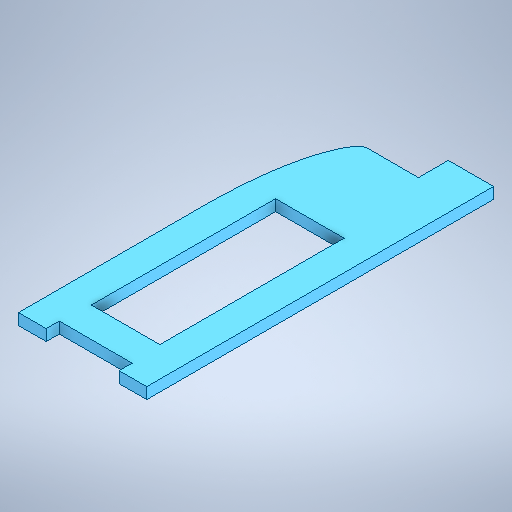
# Autodesk Inventor part: C-D
Saved by Autodesk Inventor 2025.3 (Build 293356030, 356C)
## iProperties
Created: 2025-07-09
Part Number: C-D
Material: Generic
Document SubType Name: Modeling
Designer: jv
Density: 1 g/cm^3
Appearance: Default(1)
Author: jv
Autodesk Inventor part; units mm, degrees
ref_plane "YZ Plane" through (0, 0, 0) normal (1, 0, 0) x (0, 1, 0)
ref_plane "XZ Plane" through (0, 0, 0) normal (0, 1, 0) x (-1, 0, 0)
ref_plane "XY Plane" through (0, 0, 0) normal (0, 0, 1) x (1, 0, 0)
sketch "Sketch1" plane through (0, 0, 0) normal (0, 1, 0) x (-1, 0, 0)
  line L0 (25.8082, 8) -> (28.6076, 7.9624) construction
  line L1 (0, 0) -> (0, 92.83)
  line L2 (0, 0) -> (12.1, 0)
  line L3 (26.34, 81.33) -> (8, 81.33)
  line L4 (8, 81.33) -> (8, 32)
  line L5 (8, 32) -> (26.34, 32)
  line L6 (26.34, 32) -> (26.34, 81.33)
  line L7 (0, 92.83) -> (7.42, 92.83)
  line L8 (7.42, 92.83) -> (7.42, 89.33)
  line L9 (7.42, 89.33) -> (26.92, 89.33)
  line L10 (26.92, 89.33) -> (26.92, 92.83)
  line L11 (26.92, 92.83) -> (34.34, 92.83)
  line L12 (34.34, 92.83) -> (34.34, 0)
  line L13 (34.34, 0) -> (12.1, 0)
  line L14 (12.1, 0) -> (12.1, 8)
  line L15 (12.1, 8) -> (34.34, 8)
  spline S0 degree 3 poles (25.8082, 8) (28.6076, 7.9624) (34.5101, 18.742) (34.34, 45.0104) knots 1 1 1 1 1.641396 1.641396 1.641396 1.641396
  line L16 (28.6076, 7.9624) -> (34.5101, 18.742) construction
  line L17 (34.5101, 18.742) -> (34.34, 45.0104) construction
  point P0 (25.8768, 44.3592)
  point P1 (17.17, 89.33)
  point P2 (25.8375, 8)
  point P3 (34.34, 42.8078)
  dimension "d8" = 92.83
  dimension "d9" = 12.1
  dimension "d10" = 7.42
  dimension "d11" = 7.42
  dimension "d12" = 8
  dimension "d13" = 8
  dimension "d14" = 8
  dimension "d15" = 19.5
  dimension "d16" = 3.5
  dimension "d17" = 32
  dimension "d18" = 8
  constraints: 30 end point, 7 perpendicular, 5 point on line, 3 horizontal, 2 parallel, 2 vertical, 1 coincident, 1 midpoint, 3 other
  measures "d8" distance of L1.start L1.end
  measures "d9" distance of L1.start L2.end
  measures "d10" distance of L1.end L7.end
  measures "d11" distance of L10.end L11.end
  measures "d12" distance from line of point (17.17, 89.33) L3
  measures "d13" distance between parallel lines of L12 L6
  measures "d14" distance between parallel lines of L1 L4
  measures "d15" distance of L8.end L9.end
  measures "d16" distance of L9.end L10.end
  measures "d17" distance between parallel lines of L5 L2
  measures "d18" distance of L2.end L14.end
extrude "Extrusion1" add sketch "Sketch1" along normal blind 3 contours L1 L7 L8 L9 L10 L11 L12 S0 L15 L14 L2
body "Solid1"
